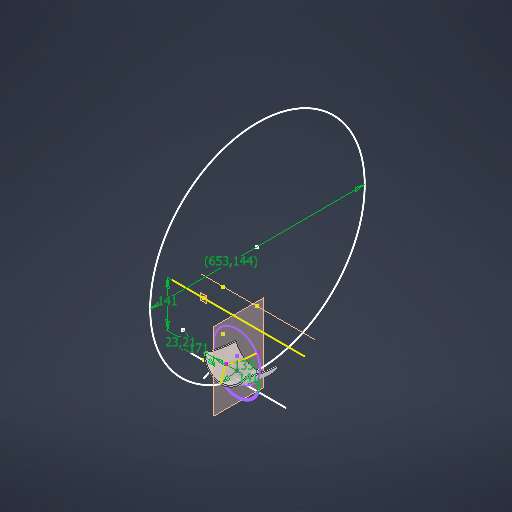
# Autodesk Inventor part: конпл направления
Saved by Autodesk Inventor 2026.2 (Build 302298000, 298)
## iProperties
Created: 2025-11-28
Part Number: конпл направления
Material: Типовые
Document SubType Name: Modeling
Designer: Phantom
Density: 1 g/cm^3
Appearance: По умолчанию
Author: Phantom
Autodesk Inventor part; units mm, degrees
ref_plane "XZ Plane" through (0, 0, 0) normal (0, 1, 0) x (-1, 0, 0)
sketch "Эскиз1" plane through (0, 0, 0) normal (0, 0, 1) x (1, 0, 0)
  arc A0 (38.6819, -124.21) -> (163.3181, -124.21) centre (101, -101) ccw
  arc A1 (34.4301, -124.21) -> (167.5699, -124.21) centre (101, -101) ccw
  line L0 (-97.5257, 0) -> (307.6841, 0) projected
  line L1 (-39.6386, -124.21) -> (244.9538, -124.21)
  point P0 (0, 0)
  point P1 (167.5699, -124.21)
  point P2 (38.6819, -124.21)
  point P3 (34.4301, -124.21)
  dimension "d0" = 133
  dimension "d1" = 141
  dimension "d3" = -101
  dimension "d4" = 23.21
  constraints: 4 point on circle, 4 point on line, 2 centre point, 2 end point, 1 coincident, 1 horizontal
  measures "d0" diameter of A0
  measures "d1" diameter of A1
  measures "d3" distance from line of A1.centre L0
  measures "d4" distance from line of L1 A0.centre
ref_plane "РабПлоскость1" through (0, 0, 60) normal (0, 0, 1) x (1, 0, 0)
sketch "Эскиз2" plane through (0, 0, 60) normal (0, 0, 1) x (1, 0, 0)
  circle A0 centre (101, -101) radius 70.5
  line L0 (-96.1046, 0) -> (307.4472, 0) projected
  arc A1 (34.4301, -164.21) -> (167.5699, -164.21) centre (101, -141) ccw
  arc A2 (38.6819, -164.21) -> (163.3181, -164.21) centre (101, -141) ccw
  line L1 (-38.4543, -164.21) -> (249.797, -164.21)
  point P0 (0, 0)
  dimension "d9" = 141
  dimension "d10" = 141
  dimension "d11" = 133
  dimension "d12" = 23.21
  constraints: 4 point on circle, 4 point on line, 3 centre point, 2 end point, 1 coincident, 1 horizontal
  measures "d9" diameter of A1
  measures "d10" distance from line of L0 A1.centre
  measures "d11" diameter of A2
  measures "d12" distance from line of A1.centre L1
sketch "Эскиз3" plane through (0, 0, 0) normal (1, 0, 0) x (0, 1, 0)
  arc A0 (-211.5, 60) -> (-171.5, 0) centre (-52.4181, 122.7213) ccw
  point P0 (0, 0)
  point P1 (-164.21, 60)
  point P2 (-124.21, 0)
  dimension "d13" = 171
  constraints: 2 point on circle, 1 centre point
  measures "d13" radius of A0
sketch "Эскиз4" plane through (0, 0, 0) normal (1, 0, 0) x (0, 1, 0)
  line L0 (0, -156.8299) -> (0, 169.3131) projected
  arc A0 (-151.3766, 110.2381) -> (-171.5, 0) centre (155.0612, -2.6563) ccw
  arc A1 (-171.3994, 5.874) -> (-171.5, 0) centre (0, 0) ccw
  point P0 (-131.3766, -110.2381)
  dimension "d25" = 326.572
  constraints: 5 point on circle, 2 centre point, 1 coincident
  measures "d25" radius of A0
sweep "Сдвиг2" add profiles "Эскиз1" path "Эскиз4" path curves A0 contours A0 L1 A1
ref_plane "РабПлоскость2" through (101, 0, 0) normal (1, 0, 0) x (0, 1, 0)
sketch "Эскиз5" plane through (101, 0, 0) normal (1, 0, 0) x (0, 1, 0)
  line L0 (-106.8707, 94.2516) -> (-106.8707, 94.2516) projected
  arc A0 (-106.8707, 94.2516) -> (-124.21, 0) centre (155.0612, -2.6563) ccw projected
  line L1 (-124.21, 0) -> (-124.21, 0) projected
  arc A1 (-106.8707, 94.2516) -> (-124.21, 0) centre (155.0612, -2.6563) ccw projected
  line L2 (-106.8707, 94.2516) -> (-106.8707, 94.2516) projected
  arc A2 (-106.8707, 94.2516) -> (-124.21, 0) centre (155.0612, -2.6563) ccw projected
  line L3 (-124.21, 0) -> (-124.21, 0) projected
  arc A3 (-106.8707, 94.2516) -> (-124.21, 0) centre (155.0612, -2.6563) ccw projected
  arc A4 (-106.8707, 94.2516) -> (-124.21, 0) centre (155.0612, -2.6563) ccw projected
  line L4 (-106.8707, 94.2516) -> (-151.3766, 110.2381) projected
  circle A5 centre (155.0612, -2.6563) radius 326.572
  point P0 (0, 0)
  dimension "d28" = 653.144
  constraints: 1 coincident, 3 other
